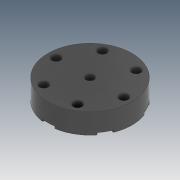
# Autodesk Inventor part: MouldTop
Saved by Autodesk Inventor 2020 (Build 240168000, 168)
## iProperties
Created: 2020-05-07
Part Number: MouldTop
Material: Generic
Document SubType Name: Modeling
Designer: Theo Cominotto
Density: 1 g/cm^3
Appearance: Default
Author: Theo Cominotto
Autodesk Inventor part; units mm, degrees
ref_plane "YZ Plane" through (0, 0, 0) normal (1, 0, 0) x (0, 1, 0)
ref_plane "XZ Plane" through (0, 0, 0) normal (0, 1, 0) x (-1, 0, 0)
ref_plane "XY Plane" through (0, 0, 0) normal (0, 0, 1) x (1, 0, 0)
sketch "Sketch1" plane through (0, 0, 0) normal (0, 0, 1) x (1, 0, 0)
  line L0 (-40, 0) -> (44, 0) construction
  line L1 (0, -7.0828) -> (0, 7.4971) construction
  line L2 (1.5, 0) -> (19, 0)
  line L3 (1.5, 0) -> (1.5, 2)
  line L4 (19, 0) -> (19, 3)
  line L5 (17, 5) -> (13, 5)
  line L6 (13, 2) -> (1.5, 2)
  line L7 (13, 2) -> (13, 5)
  line L8 (13, 2) -> (16, 2) construction
  arc A0 (19, 3) -> (17, 5) centre (17, 3) ccw
  line L9 (19, 3) -> (31, 3)
  line L10 (31, 3) -> (31, -5)
  line L11 (31, -5) -> (0, -5)
  line L12 (1.5, 2) -> (0, 2)
  line L13 (0, 2) -> (0, -5)
  line L14 (-56.8, 0) -> (60.8, 0) construction
  line L15 (0, -10.8994) -> (0, 15.8166) construction
  line L16 (31, 3) -> (31, 12)
  line L17 (31, 12) -> (0, 12)
  line L18 (0, 12) -> (0, 2)
  point P0 (0, 0)
  point P1 (0, 0)
  point P2 (19, 5)
  dimension "d0" = 19
  dimension "d1" = 1.5
  dimension "d2" = 2
  dimension "d3" = 5
  dimension "d4" = 90
  dimension "d6" = 2
  dimension "d7" = 12
  dimension "d8" = 5
  dimension "d9" = 9
  dimension "d21" = 4
  constraints: 34 end point, 6 point on line, 5 horizontal, 4 perpendicular, 4 vertical, 3 collinear, 2 point on circle, 2 tangent, 1 centre point, 3 other
  measures "d0" distance from line of L1 L4.start
  measures "d1" distance from line of L1 L2.start
  measures "d2" distance of L2.start L6.end
  measures "d3" distance of L4.start point (19, 5)
  measures "d4" angle of L8 L7
  measures "d6" radius of A0
  measures "d7" distance of L4.end L10.start
  measures "d8" distance between parallel lines of L2 L11
  measures "d9" distance of L10.start L16.end
  measures "d21" distance of L5.start L5.end
revolve "Revolution1" add sketch "Sketch1" angle 360 about axis through (0, -7.0828, 0) along (0, 1, 0) contours L12 L18 L17 L16 L9 A0 L5 L7 L6
sketch "Sketch2" plane through (0, 12, 0) normal (0, 1, 0) x (1, 0, 0)
  circle A0 centre (0, 0) radius 31 construction
  circle A1 centre (0, 0) radius 19 construction
  line L0 (-19, 0) -> (-31, 0) construction
  circle A2 centre (-25, 0) radius 3.25
  dimension "d11" = 6.5
  constraints: 2 end point, 2 horizontal alignment, 1 centre point, 1 horizontal, 1 midpoint, 2 other
  measures "d11" diameter of A2
extrude "Extrusion1" cut sketch "Sketch2" against normal up to surface (9 mm away)
pattern_circular "Circular Pattern1" count 6 over 360 about axis through (0, 7.5, 0) along (0, -1, 0) of "Extrusion1"
sketch "Sketch4" plane through (0, 0, 0) normal (0, 0, 1) x (1, 0, 0)
  line L0 (-13, 2) -> (13, 2) projected
  line L1 (0, 2) -> (0, 12)
  line L2 (-31, 12) -> (31, 12) projected
  line L3 (2.2, 2) -> (3.05, 9)
  line L4 (3.05, 9) -> (3.05, 12)
  point P0 (0, 0)
  dimension "d22" = 3.05
  dimension "d23" = 2.2
  dimension "d24" = 7
  constraints: 6 end point, 2 midpoint, 2 point on line, 1 perpendicular
  measures "d22" distance between parallel lines of L1 L4
  measures "d23" distance from line of L1 L3.start
  measures "d24" distance from line of L0 L3.end
revolve "Revolution2" cut sketch "Sketch4" angle 360 about axis through (0, 2, 0) along (0, 1, 0)
thicken "Thicken1" operation add thickness 6 both sides no extend neighbours yes toward (0, 1, 0) faces at (0.1225, 12, 14.285)
fillet "Fillet1" radius 2 1 edges at (-13, 2, 0)
fillet "Fillet2" radius 0.5 1 edges at (-13, 5, 0)
sketch "Sketch5" plane through (0, 3, 0) normal (0, -1, 0) x (1, 0, 0)
  circle A0 centre (0, 0) radius 31 projected
  circle A1 centre (0, 0) radius 3.05 construction
  line L0 (0, 0) -> (0, 31) construction
  circle A2 centre (0, 0) radius 31 construction
  line L1 (0, 0) -> (4.3144, 30.6983) construction
  line L2 (0, 0) -> (-4.3144, 30.6983) construction
  arc A3 (3.8225, 27.1983) -> (-3.8225, 27.1983) centre (0, 0) ccw
  line L3 (4.3144, 30.6983) -> (3.8225, 27.1983)
  line L4 (-3.8225, 27.1983) -> (-4.3144, 30.6983)
  point P0 (-4.3144, 30.6983)
  dimension "d30" = 8
  dimension "d31" = 3.5
  constraints: 10 end point, 2 point on circle, 2 point on line, 1 centre point, 1 coincident, 1 collinear, 1 symmetric about line, 1 vertical, 1 vertical alignment, 3 other
  measures "d30" angle of L0 L1
  measures "d31" vertical distance of L1.end L3.end
extrude "Extrusion3" cut sketch "Sketch5" against normal blind 1.5 contours L3 A3 L4 A0 picked at (-0.426, 29.7896)
chamfer "Chamfer1" distance 1.5 distance2 3.5 1 edges at (0, 4.5, 27.4656) measured on face at (0, 4, 27.4656)
fillet "Fillet3" radius 0.5 2 edges at (-4.3144, 3.75, 30.6983) (4.3144, 3.75, 30.6983)
pattern_circular "Circular Pattern2" count 6 over 360 about axis through (0, 7.5, 0) along (0, -1, 0) of "Extrusion3", "Chamfer1", "Fillet3"
body "Solid1"
